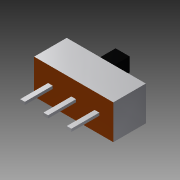
# Autodesk Inventor part: Pololu #1408 Mini Slide Switch
Saved by Autodesk Inventor 2014 SP1 (Build 180222100, 222)
## iProperties
Created: 2013-12-20
Part Number: Pololu #1408 Mini Slide Switch
Material: Generic
Document SubType Name: Modeling
Designer: JustinIndra
Density: 1 g/cm^3
Appearance: Default
Author: JustinIndra
Autodesk Inventor part; units mm, degrees
ref_plane "YZ Plane" through (0, 0, 0) normal (1, 0, 0) x (0, 1, 0)
ref_plane "XZ Plane" through (0, 0, 0) normal (0, 1, 0) x (-1, 0, 0)
ref_plane "XY Plane" through (0, 0, 0) normal (0, 0, 1) x (1, 0, 0)
sketch "Sketch1" plane through (0, 0, 0) normal (0, 1, 0) x (-1, 0, 0)
  line L0 (4.25, -1.85) -> (-4.25, -1.85)
  line L1 (-4.25, -1.85) -> (-4.25, 1.85)
  line L2 (-4.25, 1.85) -> (4.25, 1.85)
  line L3 (4.25, 1.85) -> (4.25, -1.85)
  point P0 (0, 0)
  point P1 (4.25, 0)
  point P2 (0, -1.85)
  dimension "d0" = 8.5
  dimension "d1" = 3.7
  constraints: 8 end point, 2 midpoint, 2 parallel, 1 horizontal, 1 horizontal alignment, 1 perpendicular, 1 vertical alignment
  measures "d0" distance of L1.end L2.end
  measures "d1" distance of L0.end L1.end
extrude "Extrusion1" add sketch "Sketch1" along normal blind 3.5
sketch "Sketch2" plane through (0, 0, 0) normal (0, -1, 0) x (1, 0, 0)
  line L0 (4.25, 1.85) -> (-4.25, 1.85) projected
  line L1 (-2.75, 0.15) -> (-2.25, 0.15)
  line L2 (-2.25, 0.15) -> (-2.25, -0.15)
  line L3 (-2.25, -0.15) -> (-2.75, -0.15)
  line L4 (-2.75, -0.15) -> (-2.75, 0.15)
  line L5 (-0.25, 0.15) -> (0.25, 0.15)
  line L6 (0.25, 0.15) -> (0.25, -0.15)
  line L7 (0.25, -0.15) -> (-0.25, -0.15)
  line L8 (-0.25, -0.15) -> (-0.25, 0.15)
  line L9 (2.25, 0.15) -> (2.75, 0.15)
  line L10 (2.75, 0.15) -> (2.75, -0.15)
  line L11 (2.75, -0.15) -> (2.25, -0.15)
  line L12 (2.25, -0.15) -> (2.25, 0.15)
  point P0 (0, 0)
  point P1 (-2.75, 0)
  point P2 (-2.5, 0.15)
  point P3 (-0.25, 0)
  point P4 (0, 0.15)
  point P5 (2.25, 0)
  point P6 (2.5, 0.15)
  dimension "d4" = 0.5
  dimension "d5" = 0.3
  dimension "d6" = 2.5
  dimension "d9" = 2.5
  constraints: 24 end point, 2 horizontal, 2 midpoint, 2 parallel, 1 horizontal alignment, 1 perpendicular, 20 other
  measures "d4" distance of L1.start L1.end
  measures "d5" distance of L3.end L1.start
  measures "d6" horizontal distance of point (0, 0) point (-2.5, 0.15)
  measures "d9" distance of L1.start L5.start
extrude "Extrusion2" add sketch "Sketch2" along normal blind 3
sketch "Sketch3" plane through (0, 3.5, 0) normal (0, 1, 0) x (1, 0, 0)
  line L0 (-1.8, 0.8) -> (1.8, 0.8)
  line L1 (1.8, 0.8) -> (1.8, -0.8)
  line L2 (1.8, -0.8) -> (-1.8, -0.8)
  line L3 (-1.8, -0.8) -> (-1.8, 0.8)
  point P0 (0, 0)
  point P1 (-1.8, 0)
  point P2 (0, 0.8)
  dimension "d16" = 1.6
  dimension "d17" = 3.6
  constraints: 8 end point, 2 midpoint, 2 parallel, 1 horizontal, 1 horizontal alignment, 1 perpendicular, 1 vertical alignment
  measures "d16" distance of L0.end L1.end
  measures "d17" distance of L0.start L0.end
extrude "Extrusion3" cut sketch "Sketch3" against normal blind 0.5
sketch "Sketch4" plane through (0, 3, 0) normal (0, 1, 0) x (1, 0, 0)
  line L0 (-1.8, -0.8) -> (-1.8, 0.8) projected
  line L1 (-1.75, 0.75) -> (-0.25, 0.75)
  line L2 (-0.25, 0.75) -> (-0.25, -0.75)
  line L3 (-0.25, -0.75) -> (-1.75, -0.75)
  line L4 (-1.75, -0.75) -> (-1.75, 0.75)
  point P0 (0, 0)
  point P1 (-1.75, 0)
  dimension "d20" = 1.5
  dimension "d21" = 0.05
  constraints: 8 end point, 2 parallel, 2 perpendicular, 1 horizontal, 1 horizontal alignment, 1 midpoint
  measures "d20" distance of L1.start L1.end
  measures "d21" distance between parallel lines of L0 L4
extrude "Extrusion4" add sketch "Sketch4" along normal blind 3.5
chamfer "Chamfer1" distance 0.25 angle 45 4 edges at (-1, 6.5, 0.75) (-0.25, 6.5, 0) (-1, 6.5, -0.75) (-1.75, 6.5, 0)
body "Solid1"
